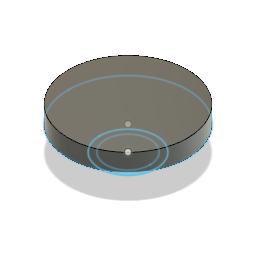
Servoattaxcher (Autodesk Fusion 360 design; units mm, degrees)
Autodesk Fusion 360 part; units mm, degrees
sketch "sketch 366" plane through (0, 33.0178, 0) normal (0, 1, 0) x (-1, 0, 0)
  circle A0 centre (-1.5233, 27.7832) radius 2.5
  circle A1 centre (-1.5233, 27.7832) radius 3.2
  circle A2 centre (-1.5233, 27.7832) radius 3.2
extrude "Extrude1" add sketch "sketch 366" along normal blind 2.5 from surface at 0.25
sketch "sketch 353" plane through (0, 35.7678, 0) normal (0, 1, 0) x (-1, 0, 0)
  circle A0 centre (-1.5233, 27.7832) radius 6.7467
extrude "Extrude2" add sketch "sketch 353" along normal blind 2
